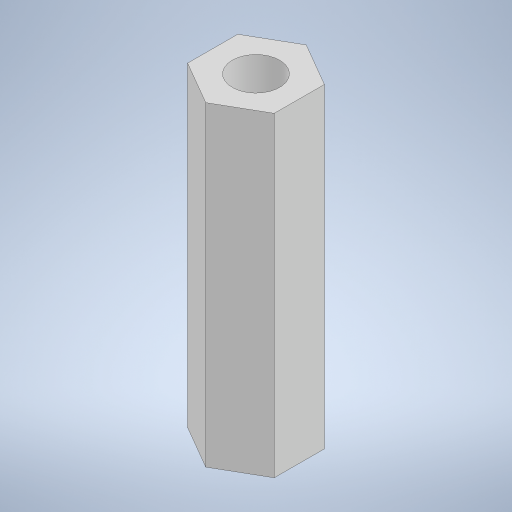
# Autodesk Inventor part: стойка
Saved by Autodesk Inventor 2023.1 (Build 271208000, 208)
## iProperties
Created: 2025-01-13
Part Number: стойка
Material: Типовые
Document SubType Name: Modeling
Designer: DELL
Density: 1 g/cm^3
Appearance: По умолчанию
Author: DELL
Autodesk Inventor part; units mm, degrees
ref_plane "YZ Plane" through (0, 0, 0) normal (1, 0, 0) x (0, 1, 0)
ref_plane "XZ Plane" through (0, 0, 0) normal (0, 1, 0) x (-1, 0, 0)
ref_plane "XY Plane" through (0, 0, 0) normal (0, 0, 1) x (1, 0, 0)
sketch "Эскиз1" plane through (0, 0, 0) normal (0, 1, 0) x (-1, 0, 0)
  line L0 (-2.7462, 1.5942) -> (0.0075, 3.1754)
  line L1 (0.0075, 3.1754) -> (2.7538, 1.5812)
  line L2 (2.7538, 1.5812) -> (2.7462, -1.5942)
  line L3 (2.7462, -1.5942) -> (-0.0075, -3.1754)
  line L4 (-0.0075, -3.1754) -> (-2.7538, -1.5812)
  line L5 (-2.7538, -1.5812) -> (-2.7462, 1.5942)
  circle A0 centre (0, 0) radius 1.5
  dimension "d0" = 5.5
  dimension "d1" = 3
  constraints: 12 end point, 2 coincident, 1 centre point, 13 other
  measures "d0" distance between parallel lines of L2 L5
  measures "d1" diameter of A0
extrude "Выдавливание1" add sketch "Эскиз1" along normal blind 20
